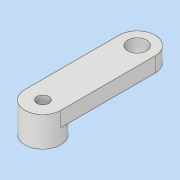
# Autodesk Inventor part: potentiometerServohornAttachment
Saved by Autodesk Inventor 2017 (Build 210142000, 142)
## iProperties
Created: 2016-12-12
Part Number: potentiometerServohornAttachment
Material: ABS Plastic
Document SubType Name: Modeling
Designer: techn
Density: 1.06 g/cm^3
Appearance: Smooth - White
Author: techn
Autodesk Inventor part; units mm, degrees
ref_plane "YZ Plane" through (0, 0, 0) normal (1, 0, 0) x (0, 1, 0)
ref_plane "XZ Plane" through (0, 0, 0) normal (0, 1, 0) x (-1, 0, 0)
ref_plane "XY Plane" through (0, 0, 0) normal (0, 0, 1) x (1, 0, 0)
sketch "Sketch1" plane through (0, 0, 0) normal (0, 1, 0) x (-1, 0, 0)
  circle A0 centre (0, 0) radius 0.635
  line L0 (0, 0) -> (0, -10)
  circle A1 centre (0, -10) radius 1
  circle A2 centre (0, -10) radius 1.905
  circle A3 centre (0, 0) radius 1.905
  line L1 (1.905, 0) -> (1.905, -10)
  line L2 (-1.905, 0) -> (-1.905, -10)
  dimension "d0" = 1.27
  dimension "d1" = 10
  dimension "d2" = 2
  dimension "d3" = 3.81
  dimension "d4" = 3.81
  constraints: 6 end point, 4 centre point, 4 coincident, 4 point on circle, 2 tangent, 2 vertical
  measures "d0" diameter of A0
  measures "d1" distance of L0.start L0.end
  measures "d2" diameter of A1
  measures "d3" diameter of A2
  measures "d4" diameter of A3
extrude "Extrusion1" add sketch "Sketch1" along normal blind 3.175
sketch "Sketch2" plane through (0, 0, 0) normal (0, -1, 0) x (1, 0, 0)
  circle A0 centre (0, 0) radius 1.905
  circle A1 centre (0, -10) radius 1 projected
  circle A2 centre (0, 0) radius 0.635 projected
  arc A3 (1.905, 0) -> (-1.905, 0) centre (0, 0) ccw projected
  line L0 (-1.905, -10) -> (-1.905, 0) projected
  arc A4 (-1.905, -10) -> (1.905, -10) centre (0, -10) ccw projected
  line L1 (1.905, 0) -> (1.905, -10) projected
  constraints: 1 centre point, 1 coincident
extrude "Extrusion2" cut sketch "Sketch2" against normal blind 1.5875 contours L1 A4 L0 A0
body "Solid1"
